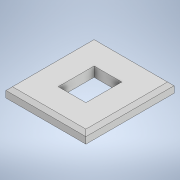
# Autodesk Inventor part: electromagnet-ending
Saved by Autodesk Inventor 2021 (Build 250183000, 183)
## iProperties
Created: 2021-01-13
Part Number: electromagnet-ending
Material: Generic
Document SubType Name: Modeling
Designer: Luke Kamols
Density: 1 g/cm^3
Appearance: Default
Author: Luke Kamols
Autodesk Inventor part; units mm, degrees
ref_plane "YZ Plane" through (0, 0, 0) normal (1, 0, 0) x (0, 1, 0)
ref_plane "XZ Plane" through (0, 0, 0) normal (0, 1, 0) x (-1, 0, 0)
ref_plane "XY Plane" through (0, 0, 0) normal (0, 0, 1) x (1, 0, 0)
sketch "Sketch1" plane through (0, 0, 0) normal (0, 1, 0) x (-1, 0, 0)
  line L0 (0, 0) -> (-8.5, 0)
  line L1 (-8.5, 0) -> (-8.5, -11)
  line L2 (-8.5, -11) -> (0, -11)
  line L3 (0, -11) -> (0, 0)
  line L4 (0, 8) -> (8, 8)
  line L5 (8, 8) -> (-16.5, 8)
  line L6 (-16.5, 8) -> (-16.5, -19)
  line L7 (-16.5, -19) -> (8, -19)
  line L8 (8, -19) -> (8, 8)
  dimension "d13" = 8.5
  dimension "d14" = 11
  dimension "d16" = 8
  dimension "d17" = 24.5
  dimension "d18" = 27
  constraints: 18 end point, 4 parallel, 2 horizontal, 2 perpendicular
  measures "d13" distance of L2.end L1.end
  measures "d14" distance of L1.end L0.end
  measures "d16" distance of L4.start L4.end
  measures "d17" distance of L7.end L6.end
  measures "d18" distance of L6.end L5.end
extrude "Extrusion1" add sketch "Sketch1" along normal blind 3
chamfer "Chamfer1" distance 1 angle 45 4 edges at (-8, 3, -5.5) (-4, 3, 8) (16.5, 3, -5.5) (4.25, 3, -19)
body "Solid1"
